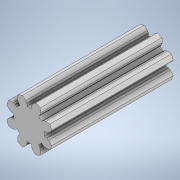
# Autodesk Inventor part: ぴにょん
Saved by Autodesk Inventor 2022.2 (Build 262287000, 287)
## iProperties
Created: 2021-11-20
Part Number: ぴにょん
Material: Generic
Document SubType Name: Modeling
Designer: muzho
Density: 1 g/cm^3
Appearance: Default
Author: muzho
Autodesk Inventor part; units mm, degrees
ref_plane "YZ Plane" through (0, 0, 0) normal (1, 0, 0) x (0, 1, 0)
ref_plane "XZ Plane" through (0, 0, 0) normal (0, 1, 0) x (-1, 0, 0)
ref_plane "XY Plane" through (0, 0, 0) normal (0, 0, 1) x (1, 0, 0)
sketch "Sketch1" plane through (0, 0, 0) normal (0, 0, 1) x (1, 0, 0)
  arc A0 (0.2626, 1.917) -> (0.2462, 1.8632) centre (0.4994, 1.8157) ccw
  arc A1 (0.3627, 2.0876) -> (0.2626, 1.917) centre (0.9307, 1.6395) ccw
  arc A2 (0.7114, 2.3967) -> (0.3627, 2.0876) centre (1.3933, 1.2761) ccw
  arc A3 (-1.1698, 1.5411) -> (-1.1434, 1.4916) centre (-0.9308, 1.637) ccw
  arc A4 (-1.2197, 1.7326) -> (-1.1698, 1.5411) centre (-0.5012, 1.8175) ccw
  arc A5 (-1.1917, 2.1977) -> (-1.2197, 1.7326) centre (0.0829, 1.8876) ccw
  arc A6 (-1.917, 0.2626) -> (-1.8632, 0.2462) centre (-1.8157, 0.4994) ccw
  arc A7 (-2.0876, 0.3627) -> (-1.917, 0.2626) centre (-1.6395, 0.9307) ccw
  arc A8 (-2.3967, 0.7114) -> (-2.0876, 0.3627) centre (-1.2761, 1.3933) ccw
  arc A9 (-1.5411, -1.1698) -> (-1.4916, -1.1434) centre (-1.637, -0.9308) ccw
  arc A10 (-1.7326, -1.2197) -> (-1.5411, -1.1698) centre (-1.8175, -0.5012) ccw
  arc A11 (-2.1977, -1.1917) -> (-1.7326, -1.2197) centre (-1.8876, 0.0829) ccw
  arc A12 (-0.2626, -1.917) -> (-0.2462, -1.8632) centre (-0.4994, -1.8157) ccw
  arc A13 (-0.3627, -2.0876) -> (-0.2626, -1.917) centre (-0.9307, -1.6395) ccw
  arc A14 (-0.7114, -2.3967) -> (-0.3627, -2.0876) centre (-1.3933, -1.2761) ccw
  arc A15 (1.1698, -1.5411) -> (1.1434, -1.4916) centre (0.9308, -1.637) ccw
  arc A16 (1.2197, -1.7326) -> (1.1698, -1.5411) centre (0.5012, -1.8175) ccw
  arc A17 (1.1917, -2.1977) -> (1.2197, -1.7326) centre (-0.0829, -1.8876) ccw
  arc A18 (1.917, -0.2626) -> (1.8632, -0.2462) centre (1.8157, -0.4994) ccw
  arc A19 (2.0876, -0.3627) -> (1.917, -0.2626) centre (1.6395, -0.9307) ccw
  arc A20 (2.3967, -0.7114) -> (2.0876, -0.3627) centre (1.2761, -1.3933) ccw
  arc A21 (1.5411, 1.1698) -> (1.4916, 1.1434) centre (1.637, 0.9308) ccw
  arc A22 (1.7326, 1.2197) -> (1.5411, 1.1698) centre (1.8175, 0.5012) ccw
  arc A23 (2.1977, 1.1917) -> (1.7326, 1.2197) centre (1.8876, -0.0829) ccw
  arc A24 (-0.2462, 1.8632) -> (-0.2626, 1.917) centre (-0.4994, 1.8157) ccw
  arc A25 (-0.2626, 1.917) -> (-0.3627, 2.0876) centre (-0.9307, 1.6395) ccw
  arc A26 (-0.3627, 2.0876) -> (-0.7114, 2.3967) centre (-1.3933, 1.2761) ccw
  arc A27 (-1.4916, 1.1434) -> (-1.5411, 1.1698) centre (-1.637, 0.9308) ccw
  arc A28 (-1.5411, 1.1698) -> (-1.7326, 1.2197) centre (-1.8175, 0.5012) ccw
  arc A29 (-1.7326, 1.2197) -> (-2.1977, 1.1917) centre (-1.8876, -0.0829) ccw
  arc A30 (-1.8632, -0.2462) -> (-1.917, -0.2626) centre (-1.8157, -0.4994) ccw
  arc A31 (-1.917, -0.2626) -> (-2.0876, -0.3627) centre (-1.6395, -0.9307) ccw
  arc A32 (-2.0876, -0.3627) -> (-2.3967, -0.7114) centre (-1.2761, -1.3933) ccw
  arc A33 (-1.1434, -1.4916) -> (-1.1698, -1.5411) centre (-0.9308, -1.637) ccw
  arc A34 (-1.1698, -1.5411) -> (-1.2197, -1.7326) centre (-0.5012, -1.8175) ccw
  arc A35 (-1.2197, -1.7326) -> (-1.1917, -2.1977) centre (0.0829, -1.8876) ccw
  arc A36 (0.2462, -1.8632) -> (0.2626, -1.917) centre (0.4994, -1.8157) ccw
  arc A37 (0.2626, -1.917) -> (0.3627, -2.0876) centre (0.9307, -1.6395) ccw
  arc A38 (0.3627, -2.0876) -> (0.7114, -2.3967) centre (1.3933, -1.2761) ccw
  arc A39 (1.4916, -1.1434) -> (1.5411, -1.1698) centre (1.637, -0.9308) ccw
  arc A40 (1.5411, -1.1698) -> (1.7326, -1.2197) centre (1.8175, -0.5012) ccw
  arc A41 (1.7326, -1.2197) -> (2.1977, -1.1917) centre (1.8876, 0.0829) ccw
  arc A42 (1.8632, 0.2462) -> (1.917, 0.2626) centre (1.8157, 0.4994) ccw
  arc A43 (1.917, 0.2626) -> (2.0876, 0.3627) centre (1.6395, 0.9307) ccw
  arc A44 (2.0876, 0.3627) -> (2.3967, 0.7114) centre (1.2761, 1.3933) ccw
  arc A45 (1.1434, 1.4916) -> (1.1698, 1.5411) centre (0.9308, 1.637) ccw
  arc A46 (1.1698, 1.5411) -> (1.2197, 1.7326) centre (0.5012, 1.8175) ccw
  arc A47 (1.2197, 1.7326) -> (1.1917, 2.1977) centre (-0.0829, 1.8876) ccw
  arc A48 (0.2162, 1.6358) -> (-0.2162, 1.6358) centre (0, 0) ccw
  arc A49 (-1.0038, 1.3095) -> (-1.3095, 1.0038) centre (0, 0) ccw
  arc A50 (-1.6358, 0.2162) -> (-1.6358, -0.2162) centre (0, 0) ccw
  arc A51 (-1.3095, -1.0038) -> (-1.0038, -1.3095) centre (0, 0) ccw
  arc A52 (-0.2162, -1.6358) -> (0.2162, -1.6358) centre (0, 0) ccw
  arc A53 (1.0038, -1.3095) -> (1.3095, -1.0038) centre (0, 0) ccw
  arc A54 (1.6358, -0.2162) -> (1.6358, 0.2162) centre (0, 0) ccw
  arc A55 (1.3095, 1.0038) -> (1.0038, 1.3095) centre (0, 0) ccw
  arc A56 (-0.7114, 2.3967) -> (-1.1917, 2.1977) centre (0, 0) ccw
  arc A57 (-2.1977, 1.1917) -> (-2.3967, 0.7114) centre (0, 0) ccw
  arc A58 (-2.3967, -0.7114) -> (-2.1977, -1.1917) centre (0, 0) ccw
  arc A59 (-1.1917, -2.1977) -> (-0.7114, -2.3967) centre (0, 0) ccw
  arc A60 (0.7114, -2.3967) -> (1.1917, -2.1977) centre (0, 0) ccw
  arc A61 (2.1977, -1.1917) -> (2.3967, -0.7114) centre (0, 0) ccw
  arc A62 (2.3967, 0.7114) -> (2.1977, 1.1917) centre (0, 0) ccw
  arc A63 (1.1917, 2.1977) -> (0.7114, 2.3967) centre (0, 0) ccw
  line L0 (0.2162, 1.6358) -> (0.2462, 1.8632)
  line L1 (-1.0038, 1.3095) -> (-1.1434, 1.4916)
  line L2 (-1.6358, 0.2162) -> (-1.8632, 0.2462)
  line L3 (-1.3095, -1.0038) -> (-1.4916, -1.1434)
  line L4 (-0.2162, -1.6358) -> (-0.2462, -1.8632)
  line L5 (1.0038, -1.3095) -> (1.1434, -1.4916)
  line L6 (1.6358, -0.2162) -> (1.8632, -0.2462)
  line L7 (1.3095, 1.0038) -> (1.4916, 1.1434)
  line L8 (-0.2162, 1.6358) -> (-0.2462, 1.8632)
  line L9 (-1.3095, 1.0038) -> (-1.4916, 1.1434)
  line L10 (-1.6358, -0.2162) -> (-1.8632, -0.2462)
  line L11 (-1.0038, -1.3095) -> (-1.1434, -1.4916)
  line L12 (0.2162, -1.6358) -> (0.2462, -1.8632)
  line L13 (1.3095, -1.0038) -> (1.4916, -1.1434)
  line L14 (1.6358, 0.2162) -> (1.8632, 0.2462)
  line L15 (1.0038, 1.3095) -> (1.1434, 1.4916)
  point P0 (1.3095, 1.0038)
  point P1 (1.0038, 1.3095)
  point P2 (1.1434, 1.4916)
  point P3 (1.1683, 1.5373)
  point P4 (1.2195, 1.7312)
  point P5 (1.1917, 2.1977)
  point P6 (0.7114, 2.3967)
  point P7 (0.3618, 2.0865)
  point P8 (0.261, 1.9131)
  point P9 (0.2462, 1.8632)
  point P10 (0.2162, 1.6358)
  point P11 (-0.2162, 1.6358)
  point P12 (-0.2462, 1.8632)
  point P13 (-0.261, 1.9131)
  point P14 (-0.3618, 2.0865)
  point P15 (-0.7114, 2.3967)
  point P16 (-1.1917, 2.1977)
  point P17 (-1.2195, 1.7312)
  point P18 (-1.1683, 1.5373)
  point P19 (-1.1434, 1.4916)
  point P20 (-1.0038, 1.3095)
  point P21 (-1.3095, 1.0038)
  point P22 (-1.4916, 1.1434)
  point P23 (-1.5373, 1.1683)
  point P24 (-1.7312, 1.2195)
  point P25 (-2.1977, 1.1917)
  point P26 (-2.3967, 0.7114)
  point P27 (-2.0865, 0.3618)
  point P28 (-1.9131, 0.261)
  point P29 (-1.8632, 0.2462)
  point P30 (-1.6358, 0.2162)
  point P31 (-1.6358, -0.2162)
  point P32 (-1.8632, -0.2462)
  point P33 (-1.9131, -0.261)
  point P34 (-2.0865, -0.3618)
  point P35 (-2.3967, -0.7114)
  point P36 (-2.1977, -1.1917)
  point P37 (-1.7312, -1.2195)
  point P38 (-1.5373, -1.1683)
  point P39 (-1.4916, -1.1434)
  point P40 (-1.3095, -1.0038)
  point P41 (-1.0038, -1.3095)
  point P42 (-1.1434, -1.4916)
  point P43 (-1.1683, -1.5373)
  point P44 (-1.2195, -1.7312)
  point P45 (-1.1917, -2.1977)
  point P46 (-0.7114, -2.3967)
  point P47 (-0.3618, -2.0865)
  point P48 (-0.261, -1.9131)
  point P49 (-0.2462, -1.8632)
  point P50 (-0.2162, -1.6358)
  point P51 (0.2162, -1.6358)
  point P52 (0.2462, -1.8632)
  point P53 (0.261, -1.9131)
  point P54 (0.3618, -2.0865)
  point P55 (0.7114, -2.3967)
  point P56 (1.1917, -2.1977)
  point P57 (1.2195, -1.7312)
  point P58 (1.1683, -1.5373)
  point P59 (1.1434, -1.4916)
  point P60 (1.0038, -1.3095)
  point P61 (1.3095, -1.0038)
  point P62 (1.4916, -1.1434)
  point P63 (1.5373, -1.1683)
  point P64 (1.7312, -1.2195)
  point P65 (2.1977, -1.1917)
  point P66 (2.3967, -0.7114)
  point P67 (2.0865, -0.3618)
  point P68 (1.9131, -0.261)
  point P69 (1.8632, -0.2462)
  point P70 (1.6358, -0.2162)
  point P71 (1.6358, 0.2162)
  point P72 (1.8632, 0.2462)
  point P73 (1.9131, 0.261)
  point P74 (2.0865, 0.3618)
  point P75 (2.3967, 0.7114)
  point P76 (2.1977, 1.1917)
  point P77 (1.7312, 1.2195)
  point P78 (1.5373, 1.1683)
  point P79 (1.4916, 1.1434)
  constraints: 128 point on circle, 64 centre point, 32 end point
extrude "Extrusion1" add sketch "Sketch1" along normal blind 13
body "Solid1"
